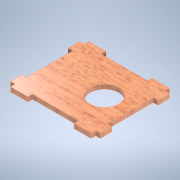
# Autodesk Inventor part: SideFemale_70wx60h
Saved by Autodesk Inventor 2022.2 (Build 262287000, 287)
## iProperties
Created: 2023-04-17
Part Number: SideFemale_70wx60h
Material: Wood (Oak)
Document SubType Name: Modeling
Designer: jaege
Density: 0.76 g/cm^3
Appearance: Red Oak - Natural Low Gloss
Author: jaege
Autodesk Inventor part; units mm, degrees
ref_plane "YZ Plane" through (0, 0, 0) normal (1, 0, 0) x (0, 1, 0)
ref_plane "XZ Plane" through (0, 0, 0) normal (0, 1, 0) x (-1, 0, 0)
ref_plane "XY Plane" through (0, 0, 0) normal (0, 0, 1) x (1, 0, 0)
sketch "Sketch1" plane through (0, 0, 0) normal (0, 1, 0) x (-1, 0, 0)
  line L0 (35, 30) -> (-35, 30) construction
  line L1 (-35, 30) -> (-35, -30) construction
  line L2 (-35, -30) -> (35, -30) construction
  line L3 (35, -30) -> (35, 30) construction
  line L4 (-35, -20) -> (-39, -20)
  line L5 (-39, -20) -> (-39, -30)
  line L6 (-39, -30) -> (-35, -30)
  line L7 (-35, -30) -> (-35, -20) construction
  line L8 (-35, 20) -> (-39, 20)
  line L9 (-39, 20) -> (-39, 30)
  line L10 (-39, 30) -> (-35, 30)
  line L11 (-35, 30) -> (-35, 20) construction
  line L12 (35, 30) -> (39, 30)
  line L13 (39, 30) -> (39, 20)
  line L14 (39, 20) -> (35, 20)
  line L15 (35, 20) -> (35, 30) construction
  line L16 (35, -30) -> (39, -30)
  line L17 (39, -30) -> (39, -20)
  line L18 (39, -20) -> (35, -20)
  line L19 (35, -20) -> (35, -30) construction
  line L20 (20, -30) -> (35, -30) construction
  line L21 (35, -30) -> (35, -34)
  line L22 (35, -34) -> (20, -34)
  line L23 (20, -34) -> (20, -30)
  line L24 (-20, -30) -> (-35, -30) construction
  line L25 (-35, -30) -> (-35, -34)
  line L26 (-35, -34) -> (-20, -34)
  line L27 (-20, -34) -> (-20, -30)
  line L28 (-35, 30) -> (-20, 30) construction
  line L29 (-20, 30) -> (-20, 34)
  line L30 (-20, 34) -> (-35, 34)
  line L31 (-35, 34) -> (-35, 30)
  line L32 (20, 34) -> (35, 34)
  line L33 (35, 34) -> (35, 30)
  line L34 (35, 30) -> (20, 30) construction
  line L35 (20, 30) -> (20, 34)
  line L36 (20, -30) -> (-20, -30)
  line L37 (-35, 20) -> (-35, -20)
  line L38 (35, -20) -> (35, 20)
  line L39 (20, 30) -> (-20, 30)
  point P0 (0, 0)
  point P1 (37, 20)
  point P2 (37, -20)
  point P3 (-20, -32)
  point P4 (20, -32)
  point P5 (0, -30)
  point P6 (35, 0)
  dimension "d0" = 70
  dimension "d1" = 60
  dimension "d2" = 4
  dimension "d3" = 40
  dimension "d4" = 40
  constraints: 80 end point, 19 parallel, 16 point on line, 10 horizontal, 10 perpendicular, 6 midpoint, 5 collinear, 5 equal length, 3 coincident, 2 horizontal alignment, 1 vertical alignment
  measures "d0" distance between parallel lines of L1 L3
  measures "d1" distance between parallel lines of L0 L2
  measures "d2" distance of L20.end L21.end
  measures "d3" distance of point (37, 20) point (37, -20)
  measures "d4" distance of point (-20, -32) point (20, -32)
extrude "Extrusion1" add sketch "Sketch1" along normal blind 4
sketch "Sketch2" plane through (0, 4, 0) normal (0, 1, 0) x (1, 0, 0)
  circle A0 centre (12.5, 0) radius 12.5
  line L0 (35, -20) -> (35, 20) projected
  point P0 (0, 0)
  dimension "d7" = 25
  dimension "d8" = 10
  constraints: 1 centre point, 1 horizontal alignment
  measures "d7" diameter of A0
  measures "d8" distance edge to line of A0 L0
extrude "Extrusion2" cut sketch "Sketch2" against normal blind 4
body "Solid1"
